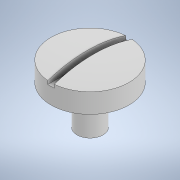
# Autodesk Inventor part: Ch7(5) Part 12 Screw NEED TO DO
Saved by Autodesk Inventor 2020 (Build 240168000, 168)
## iProperties
Created: 2021-03-04
Part Number: Ch7(5) Part 12 Screw NEED TO DO
Material: Generic
Document SubType Name: Modeling
Designer: adriggs
Density: 1 g/cm^3
Appearance: Default
Author: adriggs
Autodesk Inventor part; units mm, degrees
ref_plane "YZ Plane" through (0, 0, 0) normal (1, 0, 0) x (0, 1, 0)
ref_plane "XZ Plane" through (0, 0, 0) normal (0, 1, 0) x (-1, 0, 0)
ref_plane "XY Plane" through (0, 0, 0) normal (0, 0, 1) x (1, 0, 0)
sketch "Sketch1" plane through (0, 0, 0) normal (0, 0, 1) x (1, 0, 0)
  line L0 (0, 0) -> (19.05, 0)
  line L1 (-9.525, 9.4996) -> (9.525, 9.4996)
  line L2 (-9.525, 9.4996) -> (-9.525, 14.2748)
  line L3 (-9.525, 14.2748) -> (9.525, 14.2748)
  line L4 (9.525, 14.2748) -> (9.525, 9.4996)
  line L5 (0, 14.2748) -> (0, 15.8496)
  arc A0 (9.525, 14.2748) -> (-9.525, 14.2748) centre (0, -13.7432) ccw
  line L6 (0, 9.4996) -> (0, 0)
  line L7 (3.175, 0) -> (3.175, 9.4996)
  line L8 (3.175, 0) -> (-3.175, 0)
  line L9 (-3.175, 0) -> (-3.175, 9.4996)
  line L10 (-15.24, 0) -> (24.765, 0) projected
  line L11 (0, -19.6618) -> (0, 21.7682) projected
  dimension "d1" = 19.05
  dimension "d2" = 4.7752
  dimension "d4" = 1.5748
  dimension "d5" = 9.4996
  dimension "d6" = 3.175
  dimension "d7" = 6.35
  constraints: 20 end point, 4 perpendicular, 3 horizontal, 3 midpoint, 3 point on circle, 3 vertical, 2 point on line, 2 vertical alignment, 1 centre point, 1 coincident, 1 other
  measures "d1" distance of L1.start L1.end
  measures "d2" distance of L1.start L2.end
  measures "d4" distance of L5.start L5.end
  measures "d5" distance of L6.start L6.end
  measures "d6" distance of L6.end L7.start
  measures "d7" distance of L7.start L8.end
revolve "Revolution1" add sketch "Sketch1" angle 360 about axis through (0, -10, 0) along (0, 1, 0) picked at (5.3129, 14.5653) contours L6 L1 L7 L0 | L11 L3 L4 L1 | L5 A0 L3
ref_plane "Work Plane1" through (0, 15.8496, 0) normal (0, -1, 0) x (1, 0, 0)
sketch "Sketch2" plane through (0, 15.8496, 0) normal (0, -1, 0) x (1, 0, 0)
  circle A0 centre (0, 0) radius 9.525 projected
  line L0 (0.7874, 9.4924) -> (0.7874, -9.4924)
  line L1 (-0.7874, 9.4924) -> (-0.7874, -9.4924)
  line L2 (0, -13.335) -> (0, 13.335) projected
  line L3 (-13.335, 0) -> (13.335, 0) projected
  point P0 (0, 9.525)
  dimension "d11" = 1.5748
  constraints: 5 point on circle, 4 end point, 1 vertical, 1 vertical alignment, 1 other
  measures "d11" distance between parallel lines of L1 L0
extrude "Extrusion1" cut sketch "Sketch2" along normal blind 2.3876 contours L0 L3 L2 A0 | A0 L2 L3 L0 | L2 L3 L1 A0 | A0 L1 L3 L2
body "Solid1"
